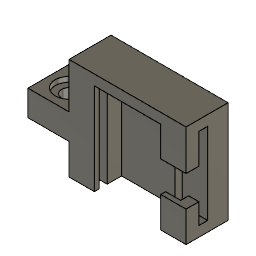
ToF_Holder (Autodesk Fusion 360 design; units mm, degrees)
Autodesk Fusion 360 part; units mm, degrees
sketch "Sketch1" plane through (0, 0, 0) normal (0, 1, 0) x (1, 0, 0)
  line L0 (0, 0) -> (22.8, 0)
  line L1 (22.8, 0) -> (22.8, -19.85)
  line L2 (22.8, -19.85) -> (0, -19.85)
  line L3 (0, -19.85) -> (0, 0)
  dimension "d8" = 19.85
  dimension "d9" = 22.8
  constraint horizontal L0
  constraint vertical L1
  constraint horizontal L2
  constraint vertical L3
  constraint coincident L0.start L3.end
  measures "d8" distance of L0.start L2.end
  measures "d9" distance of L1.end L2.end
extrude "Extrude1" add sketch "Sketch1" along normal blind 3
sketch "Sketch2" plane through (0, 0, 0) normal (0, 1, 0) x (1, 0, 0)
  circle A0 centre (6.5, -15.16) radius 0.875
  circle A1 centre (6.5, -2.5) radius 0.875
  line L0 (0, -19.85) -> (0, 0)
  line L1 (0, 0) -> (22.8, 0)
  dimension "d3" = 1.75
  dimension "d4" = 1.75
  dimension "d5" = 12.66
  dimension "d6" = 6.5
  dimension "d7" = 2.5
  constraint vertical A0.centre A1.centre
  measures "d3" diameter of A0
  measures "d4" diameter of A1
  measures "d5" distance of A0.centre A1.centre
  measures "d6" distance of A0.centre L0
  measures "d7" distance of A1.centre L1
sketch "Sketch4" plane through (0, 0, 0) normal (0, -1, 0) x (1, 0, 0)
  line L0 (22.8, 19.85) -> (0, 19.85)
  line L1 (0, 19.85) -> (0, 0)
  line L2 (0, 0) -> (22.8, 0)
  line L3 (22.8, 0) -> (22.8, 19.85)
  line L4 (0, 19.85) -> (4.95, 19.85)
  line L5 (4.95, 19.85) -> (4.95, 0)
  line L6 (4.95, 0) -> (0, 0)
  line L7 (0, 0) -> (0, 19.85)
  line L8 (22.8, 19.85) -> (17.85, 19.85)
  line L9 (17.85, 19.85) -> (17.85, 0)
  line L10 (17.85, 0) -> (22.8, 0)
  line L11 (22.8, 0) -> (22.8, 19.85)
  dimension "d12" = 4.95
  dimension "d13" = 4.95
  constraint horizontal L4
  constraint vertical L5
  constraint horizontal L6
  constraint vertical L7
  constraint coincident L2 L5.end
  constraint coincident L0.end L1.start
  constraint horizontal L8
  constraint vertical L9
  constraint horizontal L10
  constraint vertical L11
  constraint coincident L2 L9.end
  constraint coincident L0.start L3.end
  measures "d12" distance of L5 L7
  measures "d13" distance of L9 L11
extrude "Extrude3" add sketch "Sketch4" along normal blind 5.2 contours L0 L2 L3 L8 L9 L10 L11 | L0 L1 L2 L4 L5 L6 L7
sketch "Sketch5" plane through (0, 0, 19.85) normal (0, 0, 1) x (-1, 0, 0)
  line L0 (-22.8, 5.2) -> (-22.8, -3)
  line L1 (-22.8, -3) -> (0, -3)
  line L2 (0, -3) -> (0, 5.2)
  line L3 (0, 5.2) -> (-4.95, 5.2)
  line L4 (-4.95, 5.2) -> (-4.95, 0)
  line L5 (-4.95, 0) -> (-17.85, 0)
  line L6 (-17.85, 0) -> (-17.85, 5.2)
  line L7 (-17.85, 5.2) -> (-22.8, 5.2)
  line L8 (-2, 4.25) -> (-20.8, 4.25)
  line L9 (-20.8, 4.25) -> (-20.8, 2.7)
  line L10 (-20.8, 2.7) -> (-2, 2.7)
  line L11 (-2, 2.7) -> (-2, 4.25)
  dimension "d16" = 2
  dimension "d17" = 2.7
  dimension "d18" = 1.55
  dimension "d19" = 2
  constraint horizontal L8
  constraint vertical L9
  constraint horizontal L10
  constraint vertical L11
  measures "d16" distance of L2 L11
  measures "d17" distance of L5 L10
  measures "d18" distance of L8 L10
  measures "d19" distance of L0 L9
extrude "Extrude4" cut sketch "Sketch5" against normal blind 21 contours L4 L6 L8 L10 | L6 L8 L9 L10 | L4 L8 L10 L11
sketch "Sketch6" plane through (0, 0, 0) normal (0, -1, 0) x (1, 0, 0)
  line L0 (17.85, 0) -> (17.85, 19.85)
  line L1 (17.85, 19.85) -> (4.95, 19.85)
  line L2 (4.95, 19.85) -> (4.95, 0)
  line L3 (4.95, 0) -> (17.85, 0)
  line L4 (17.85, 19.85) -> (15.35, 19.85)
  line L5 (15.35, 19.85) -> (15.35, 0)
  line L6 (15.35, 0) -> (17.85, 0)
  line L7 (17.85, 0) -> (17.85, 19.85)
  dimension "d22" = 2.5
  constraint horizontal L4
  constraint vertical L5
  constraint horizontal L6
  constraint vertical L7
  constraint coincident L3 L5.end
  constraint coincident L0.end L1.start
  measures "d22" distance of L0.end L4.end
extrude "Extrude5" cut sketch "Sketch6" against normal blind 1.5 contours L0 L1 L3 L4 L5 L6 L7
sketch "Sketch7" plane through (17.85, 0, 0) normal (-1, 0, 0) x (0, -1, 0)
  line L0 (2.7, 0) -> (2.7, 19.85)
  line L1 (2.7, 19.85) -> (-1.5, 19.85)
  line L2 (-1.5, 19.85) -> (-1.5, 0)
  line L3 (-1.5, 0) -> (2.7, 0)
  line L4 (2.7, 19.85) -> (1, 19.85)
  line L5 (1, 19.85) -> (1, 2)
  line L6 (1, 2) -> (2.7, 2)
  line L7 (2.7, 2) -> (2.7, 19.85)
  dimension "d25" = 2.5
  dimension "d26" = 2
  dimension "d27" = 1.7
  constraint horizontal L4
  constraint vertical L5
  constraint horizontal L6
  constraint vertical L7
  constraint coincident L1 L0.end
  measures "d25" distance of L2 L5
  measures "d26" distance of L3 L6
  measures "d27" distance of L5 L7
extrude "Extrude6" cut sketch "Sketch7" against normal blind 13 contours L0 L1 L4 L5 L6 L7
sketch "Sketch8" plane through (0, -5.2, 0) normal (0, -1, 0) x (1, 0, 0)
  line L0 (0, 0) -> (4.95, 0)
  line L1 (4.95, 0) -> (4.95, 19.85)
  line L2 (4.95, 19.85) -> (0, 19.85)
  line L3 (0, 19.85) -> (0, 0)
  line L4 (0, 19.85) -> (22.8, 19.85)
  line L5 (22.8, 19.85) -> (22.8, 17.85)
  line L6 (22.8, 17.85) -> (0, 17.85)
  line L7 (0, 17.85) -> (0, 19.85)
  dimension "d30" = 2
  dimension "d31" = 22.8
  constraint horizontal L4
  constraint vertical L5
  constraint horizontal L6
  constraint vertical L7
  constraint coincident L2.end L3.start
  measures "d30" distance of L2.end L6.end
  measures "d31" distance of L5.end L6.end
extrude "Extrude7" add sketch "Sketch8" against normal blind 8 contours L1 L2 L3 L4 L6 L7 | L1 L4 L5 L6
sketch "Sketch9" plane through (0, -5.2, 0) normal (0, -1, 0) x (1, 0, 0)
  line L0 (17.85, 17.85) -> (17.85, 0)
  line L1 (17.85, 0) -> (22.8, 0)
  line L2 (22.8, 0) -> (22.8, 19.85)
  line L3 (22.8, 19.85) -> (0, 19.85)
  line L4 (0, 19.85) -> (0, 0)
  line L5 (0, 0) -> (4.95, 0)
  line L6 (4.95, 0) -> (4.95, 17.85)
  line L7 (4.95, 17.85) -> (17.85, 17.85)
  line L8 (17.85, 6) -> (22.8, 6)
  line L9 (22.8, 6) -> (22.8, 12)
  line L10 (22.8, 12) -> (17.85, 12)
  line L11 (17.85, 12) -> (17.85, 6)
  dimension "d34" = 6
  dimension "d35" = 6
  constraint horizontal L8
  constraint vertical L9
  constraint horizontal L10
  constraint vertical L11
  constraint coincident L2 L9.end
  constraint coincident L0 L8.start
  measures "d34" distance of L8 L10
  measures "d35" distance of L1 L8
extrude "Extrude8" cut sketch "Sketch9" against normal blind 3 contours L0 L2 L8 L9 L10 L11
sketch "Sketch10" plane through (0, 0, 0) normal (-1, 0, 0) x (0, -1, 0)
  line L0 (5.2, 19.85) -> (-3, 19.85)
  line L1 (-3, 19.85) -> (-3, 0)
  line L2 (-3, 0) -> (5.2, 0)
  line L3 (5.2, 0) -> (5.2, 19.85)
  line L4 (-3, 11) -> (5.2, 11)
  line L5 (5.2, 11) -> (5.2, 6)
  line L6 (5.2, 6) -> (-3, 6)
  line L7 (-3, 6) -> (-3, 11)
  dimension "d38" = 5
  dimension "d39" = 6
  constraint horizontal L4
  constraint vertical L5
  constraint horizontal L6
  constraint vertical L7
  constraint coincident L3 L5.end
  constraint coincident L1 L4.start
  measures "d38" distance of L4 L6
  measures "d39" distance of L2 L6
extrude "Extrude9" add sketch "Sketch10" along normal blind 8 contours L1 L3 L4 L5 L6 L7
sketch "Sketch11" plane through (0, 0, 11) normal (0, 0, 1) x (-1, 0, 0)
  line L0 (0, 5.2) -> (0, -3)
  line L1 (0, -3) -> (8, -3)
  line L2 (8, -3) -> (8, 5.2)
  line L3 (8, 5.2) -> (0, 5.2)
  circle A0 centre (4, 1.1) radius 2.75
  dimension "d42" = 4.1
  dimension "d43" = 4
  dimension "d44" = 5.5
  measures "d42" distance of L1 A0.centre
  measures "d43" distance of L2 A0.centre
  measures "d44" diameter of A0
extrude "Extrude10" cut sketch "Sketch11" against normal blind 1 contours A0
sketch "Sketch12" plane through (0, 0, 10) normal (0, 0, 1) x (-1, 0, 0)
  circle A0 centre (4, 1.1) radius 2.75
  circle A1 centre (4, 1.1) radius 1.5
  dimension "d47" = 3
  constraint concentric A0 A1
  measures "d47" diameter of A1
extrude "Extrude11" cut sketch "Sketch12" against normal blind 4 contours A1
sketch "Sketch13" plane through (0, 0, 0) normal (0, -1, 0) x (1, 0, 0)
  line L0 (15.35, 17.85) -> (4.95, 17.85)
  line L1 (4.95, 17.85) -> (4.95, 0)
  line L2 (4.95, 0) -> (15.35, 0)
  line L3 (15.35, 0) -> (15.35, 17.85)
  line L4 (15.35, 17.85) -> (4.95, 17.85)
  line L5 (4.95, 17.85) -> (4.95, 0)
  line L6 (4.95, 0) -> (15.35, 0)
  line L7 (15.35, 0) -> (15.35, 17.85)
  constraint horizontal L4
  constraint vertical L5
  constraint horizontal L6
  constraint vertical L7
  constraint coincident L1.end L2.start
  constraint coincident L0.start L3.end
extrude "Extrude12" cut sketch "Sketch13" against normal blind 0.1
equation "d14 = 2.5 mm + 2.7 mm"
